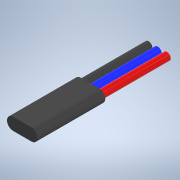
# Autodesk Inventor part: SLEEVE
Saved by Autodesk Inventor 2022 (Build 260153000, 153)
## iProperties
Created: 2022-07-28
Part Number: SLEEVE
Material: Rubber, Silicone
Document SubType Name: Modeling
Designer: Nathan Cai
Density: 1.25 g/cm^3
Appearance: Rubber - Black
Author: Nathan Cai
Autodesk Inventor part; units mm, degrees
ref_plane "YZ Plane" through (0, 0, 0) normal (1, 0, 0) x (0, 1, 0)
ref_plane "XZ Plane" through (0, 0, 0) normal (0, 1, 0) x (-1, 0, 0)
ref_plane "XY Plane" through (0, 0, 0) normal (0, 0, 1) x (1, 0, 0)
sketch "Sketch1" plane through (0, 0, 0) normal (0, 0, 1) x (1, 0, 0)
  line L0 (-3, 0) -> (3, 0) construction
  line L1 (-3, -2) -> (3, -2)
  line L2 (3, 2) -> (-3, 2)
  arc A0 (-3, 2) -> (-3, -2) centre (-3, 0) ccw
  arc A1 (3, -2) -> (3, 2) centre (3, 0) ccw
  point P0 (0, 0)
  dimension "d0" = 4
  dimension "d1" = 6
  constraints: 8 end point, 4 point on circle, 4 tangent, 2 centre point, 1 horizontal, 1 midpoint, 1 parallel
  measures "d0" diameter of A1
  measures "d1" distance of L0.start L0.end
extrude "Extrusion1" add sketch "Sketch1" along normal blind 22.225
sketch "Sketch2" plane through (0, 0, 0) normal (0, 0, -1) x (-1, 0, 0)
  circle A0 centre (0, 0) radius 1.25
  circle A1 centre (-3, 0) radius 1.25
  arc A2 (-3, 2) -> (-3, -2) centre (-3, 0) ccw projected
  circle A3 centre (3, 0) radius 1.25
  dimension "d4" = 2.5
  dimension "d5" = 2.5
  dimension "d8" = 360
  constraints: 3 centre point, 1 coincident, 1 concentric, 5 other
  measures "d4" diameter of A0
  measures "d5" diameter of A1
extrude "Extrusion2" add sketch "Sketch2" along normal blind 22.225
body "Solid1"
